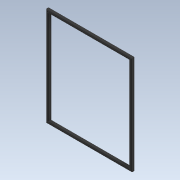
# Autodesk Inventor part: Dichtung_final
Saved by Autodesk Inventor 2020 (Build 240168000, 168)
## iProperties
Created: 2022-02-08
Part Number: Dichtung_final
Material: Gummi
Document SubType Name: Modeling
Designer: Julian Uhl
Density: 0.93 g/cm^3
Appearance: Gummi - Schwarz
Author: Julian Uhl
Autodesk Inventor part; units mm, degrees
ref_plane "YZ Plane" through (0, 0, 0) normal (1, 0, 0) x (0, 1, 0)
ref_plane "XZ Plane" through (0, 0, 0) normal (0, 1, 0) x (-1, 0, 0)
ref_plane "XY Plane" through (0, 0, 0) normal (0, 0, 1) x (1, 0, 0)
sketch "Skizze1" plane through (0, 0, 0) normal (0, 0, 1) x (1, 0, 0)
  line L0 (0, 0) -> (98, 0)
  line L1 (98, 0) -> (98, 113)
  line L2 (98, 113) -> (0, 113)
  line L3 (0, 113) -> (0, 0)
  line L4 (3, 3) -> (95, 3)
  line L5 (95, 3) -> (95, 110)
  line L6 (95, 110) -> (3, 110)
  line L7 (3, 110) -> (3, 3)
  dimension "d0" = 107
  dimension "d1" = 92
  dimension "d2" = 98
  dimension "d3" = 113
  dimension "d4" = 3
  dimension "d5" = 3
  constraints: 16 end point, 4 parallel, 2 horizontal, 2 perpendicular
  measures "d0" distance between parallel lines of L4 L6
  measures "d1" distance between parallel lines of L5 L7
  measures "d2" distance between parallel lines of L3 L1
  measures "d3" distance between parallel lines of L0 L2
  measures "d4" distance between parallel lines of L0 L4
  measures "d5" distance between parallel lines of L3 L7
extrude "Extrusion1" add sketch "Skizze1" along normal blind 3
fillet "Rundung1" radius 1 8 edges at (3, 56.5, 3) (0, 56.5, 3) (49, 110, 3) (49, 113, 3) (98, 56.5, 3) (95, 56.5, 3) (49, 0, 3) (49, 3, 3)
